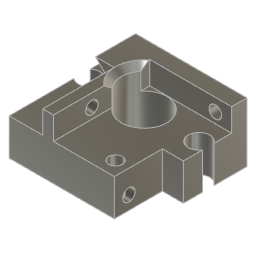
hotswap mx solderable v5 (Autodesk Fusion 360 design; units mm, degrees)
Autodesk Fusion 360 part; units mm, degrees
note: some values were not read from the file. Chosen so that the rebuilt part matches the saved one: which bodies a step acts on; which face or edge a step refers to. Set by a fixed rule: which sketch regions a step uses.
sketch "body" plane through (0, 0, 0) normal (0, 0, 1) x (1, 0, 0)
  circle A0 centre (0, 0) radius 2
  circle A1 centre (4.8, 0) radius 0.95
  circle A2 centre (-4.8, 0) radius 0.95
  circle A3 centre (2.6, -5.1) radius 0.6
  circle A4 centre (-3.8, -2.5) radius 0.6
  line L0 (-5.426, 3.3769) -> (5.6055, 3.3769)
  line L1 (5.6055, 3.3769) -> (5.6055, -6.3722)
  line L2 (5.6055, -6.3722) -> (-5.426, -6.3722)
  line L3 (-5.426, -6.3722) -> (-5.426, 3.3769)
  line L4 (5.6055, -6.3722) -> (3.771, -6.3722)
  line L5 (3.771, -6.3722) -> (3.771, -2.1749)
  line L6 (3.771, -2.1749) -> (5.6055, -2.1749)
  line L7 (5.6055, -2.1749) -> (5.6055, -6.3722)
  line L8 (-5.426, 3.3769) -> (-8.926, 3.3769)
  line L9 (-8.926, 3.3769) -> (-8.926, -1.5107)
  line L10 (-8.926, -1.5107) -> (-5.426, -1.5107)
  line L11 (-5.426, -1.5107) -> (-5.426, 3.3769)
  line L12 (5.6055, 3.3769) -> (9.1055, 3.3769)
  line L13 (9.1055, 3.3769) -> (9.1055, -1.4945)
  line L14 (9.1055, -1.4945) -> (5.6055, -1.4945)
  line L15 (5.6055, -1.4945) -> (5.6055, 3.3769)
  line L16 (-8.926, -1.5107) -> (-7.426, -1.5107)
  line L17 (-7.426, -1.5107) -> (-7.426, -5.9318)
  line L18 (-7.426, -5.9318) -> (-8.926, -5.9318)
  line L19 (-8.926, -5.9318) -> (-8.926, -1.5107)
  line L20 (9.1055, -1.4945) -> (7.6055, -1.4945)
  line L21 (7.6055, -1.4945) -> (7.6055, -5.9318)
  line L22 (7.6055, -5.9318) -> (9.1055, -5.9318)
  line L23 (9.1055, -5.9318) -> (9.1055, -1.4945)
  line L24 (6.7444, -1.4945) -> (6.7444, 3.3769)
  line L25 (-6.3235, -1.5107) -> (-6.3235, 3.3769)
  dimension "d1" = 4
  dimension "d2" = 1.9
  dimension "d3" = 1.9
  dimension "d4" = 4.8
  dimension "d5" = 4.8
  dimension "d6" = 1.2
  dimension "d7" = 1.2
  dimension "d8" = 3.8
  dimension "d9" = 2.5
  dimension "d10" = 5.1
  dimension "d11" = 2.6
  dimension "d84" = 6.3722
  dimension "d85" = 5.426
  dimension "d95" = 3.5
  dimension "d96" = 3.5
  dimension "d103" = 1.5
  dimension "d104" = 1.5
  constraint coincident A0.centre origin
  constraint horizontal L0
  constraint vertical L1
  constraint horizontal L2
  constraint vertical L3
  constraint horizontal L4
  constraint vertical L5
  constraint horizontal L6
  constraint vertical L7
  constraint horizontal A0.centre A2.centre
  constraint horizontal A0.centre A1.centre
  constraint horizontal L8
  constraint vertical L9
  constraint horizontal L10
  constraint vertical L11
  constraint horizontal L12
  constraint vertical L13
  constraint horizontal L14
  constraint vertical L15
  constraint horizontal L16
  constraint vertical L17
  constraint horizontal L18
  constraint vertical L19
  constraint horizontal L20
  constraint vertical L21
  constraint horizontal L22
  constraint vertical L23
  constraint coincident L17.end L22
  constraint coincident L14 L24.start
  constraint coincident L12 L24.end
  constraint perpendicular L12 L24
  constraint coincident L8 L25.end
  constraint perpendicular L8 L25
  constraint coincident L10 L25.start
  measures "d1" diameter of A0
  measures "d2" diameter of A1
  measures "d3" diameter of A2
  measures "d4" horizontal distance of A0.centre A2.centre
  measures "d5" horizontal distance of A0.centre A1.centre
  measures "d6" diameter of A3
  measures "d7" diameter of A4
  measures "d8" horizontal distance of A0.centre A4.centre
  measures "d9" vertical distance of A0.centre A4.centre
  measures "d10" vertical distance of A0.centre A3.centre
  measures "d11" horizontal distance of A0.centre A3.centre
  measures "d84" distance of A0.centre L2
  measures "d85" distance of A0.centre L3
  measures "d95" distance of L0.start L8.end
  measures "d96" distance of L0.end L12.end
  measures "d103" distance of L9.end L16.end
  measures "d104" distance of L13.end L20.end
extrude "Extrude1" add sketch "body" along normal blind 3.2 contours A1 L1 L12 L14 L15 L24 | A1 A2 L0 L1 L2 L3 L5 L6 L11 L15 | A2 L3 L8 L10 L11 L25 | L12 L13 L14 L20 L24 | L8 L9 L10 L16 L25 | L14 L20 L21 L22 L23 | L10 L16 L17 L18 L19 makes body 1
sketch "side holes" plane through (0, 0, 0) normal (1, 0, 0) x (0, 1, 0)
  circle A0 centre (-5.1, 1.1729) radius 0.55
  circle A1 centre (-2.5, 1.1388) radius 0.55
  point P0 (-2.5, 0)
  point P1 (-5.1, 0)
  dimension "d14" = 1.1
  dimension "d15" = 1.1
  constraint vertical P1 A0.centre
  constraint vertical P0 A1.centre
  measures "d14" diameter of A0
  measures "d15" diameter of A1
extrude "Extrude2" cut sketch "side holes" along normal up to surface (9.197 mm away) from surface at -5.426 bodies 1
sketch "2nd layer" plane through (0, 0, 3.2) normal (0, 0, 1) x (-1, 0, 0)
  circle A0 centre (3.8, 2.5) radius 0.6
  circle A1 centre (0, 0) radius 2
  circle A2 centre (-2.6, 5.1) radius 0.6
  line L0 (-3.771, 6.3722) -> (-3.771, 2.1749)
  line L1 (-3.771, 2.1749) -> (-5.6055, 2.1749)
  line L2 (-5.6055, 2.1749) -> (-5.6055, 1.4945)
  line L3 (-9.1055, -3.3769) -> (8.926, -3.3769)
  line L4 (5.426, 1.5107) -> (5.426, 6.3722)
  line L5 (5.426, 6.3722) -> (-3.771, 6.3722)
  line L6 (-9.1055, -3.3769) -> (-2.7206, -3.3769)
  line L7 (-9.1055, -0.9358) -> (-9.1055, -3.3769)
  line L8 (-5.6055, -2.0433) -> (1.5542, -2.0433)
  line L9 (1.5542, -2.0433) -> (1.5542, -3.3769)
  line L10 (1.5542, -3.3769) -> (-5.6055, -3.3769)
  line L11 (-5.6055, -3.3769) -> (-5.6055, -2.0433)
  line L12 (5.426, -3.3769) -> (4.4901, -3.3769)
  line L13 (4.4901, -3.3769) -> (4.4901, 6.3722)
  line L14 (4.4901, 6.3722) -> (5.426, 6.3722)
  line L15 (5.426, 6.3722) -> (5.426, -3.3769)
  line L16 (1.5542, 6.3722) -> (2.4901, 6.3722)
  line L17 (2.4901, 6.3722) -> (2.4901, -3.3769)
  line L18 (2.4901, -3.3769) -> (1.5542, -3.3769)
  line L19 (1.5542, -3.3769) -> (1.5542, 6.3722)
  line L20 (-9.1055, -3.3769) -> (8.926, -3.3769)
  line L21 (-2.7206, -3.3769) -> (-2.7206, -2.0433)
  line L22 (2.4901, 1.7119) -> (1.5542, 1.7119)
  circle A3 centre (-4.8, 0) radius 0.95
  circle A4 centre (4.8, 0) radius 0.95
  line L23 (-5.6055, 1.4945) -> (-7.6055, 1.4945)
  line L24 (-9.1055, 5.9318) -> (-9.1055, -3.3769)
  line L25 (8.926, -3.3769) -> (8.926, 5.9318)
  line L26 (7.426, 1.5107) -> (5.426, 1.5107)
  line L27 (5.426, 6.3722) -> (-3.771, 6.3722)
  line L28 (-7.6055, 1.4945) -> (-7.6055, 5.9318)
  line L29 (-7.6055, 5.9318) -> (-9.1055, 5.9318)
  line L30 (8.926, 5.9318) -> (7.426, 5.9318)
  line L31 (7.426, 5.9318) -> (7.426, 1.5107)
  dimension "d39" = 2
  constraint horizontal L6
  constraint vertical L7
  constraint coincident L3.start L6.start
  constraint horizontal L8
  constraint vertical L9
  constraint horizontal L10
  constraint vertical L11
  constraint horizontal L12
  constraint vertical L13
  constraint horizontal L14
  constraint vertical L15
  constraint coincident L4 L12.start
  constraint horizontal L16
  constraint vertical L17
  constraint horizontal L18
  constraint vertical L19
  constraint equal L14 L16
  constraint coincident L18 L3.end
  constraint coincident L12 L3.end
  constraint coincident L9 L16.start
  constraint coincident L10 L6.end
  constraint coincident L8 L21.end
  constraint perpendicular L8 L21
  constraint coincident L17 L22.start
  constraint coincident L19 L22.end
  constraint perpendicular L19 L22
  constraint coincident L6.end L21.start
  measures "d39" distance of L13 L17
extrude "Extrude3" add sketch "2nd layer" along normal blind 2 contours A1 L3 L9 L17 L18 L19 L20 L22 | L5 L16 L17 L19 L22 L27 | L3 L8 L9 L10 L19 L20 L21 | L3 L6 L8 L10 L11 L20 L21 bodies 1
sketch "diode fitting" plane through (0, 0, 0) normal (0, 1, 0) x (1, 0, 0)
  circle A0 centre (4.1902, -4.093) radius 0.55
  dimension "d21" = 1.1
  measures "d21" diameter of A0
extrude "Extrude4" cut sketch "diode fitting" against normal up to surface (5.5518 mm away) from surface at 3.3769 bodies 1
sketch "side hole for second layer" plane through (0, 0, 0) normal (1, 0, 0) x (0, 1, 0)
  circle A0 centre (-3.011, 4.093) radius 0.55
  point P0 (-2.5, 1.1388)
  dimension "d25" = 1.1
  measures "d25" diameter of A0
extrude "Extrude5" cut sketch "side hole for second layer" along normal up to surface (3.8718 mm away) from surface at -5.426 bodies 1
extrude "Extrude6" add sketch "side holes" against normal blind 1 from surface at 3.771 contours A1 bodies 1
extrude "Extrude7" add sketch "side holes" along normal blind 1.626 from surface at -5.426 contours A0 bodies 1
sketch "Sketch6" plane through (0, 0, 3.2) normal (0, 0, 1) x (-1, 0, 0)
  line L0 (1.5542, 6.3722) -> (-3.771, 6.3722)
  line L1 (-3.771, 6.3722) -> (-3.771, 2.1749)
  line L2 (-5.6055, -2.0433) -> (1.5542, -2.0433)
  circle A0 centre (-2.6, 5.1) radius 0.6
  line L3 (5.426, -3.3769) -> (-9.1055, -3.3769)
  line L4 (-9.1055, -3.3769) -> (-9.1055, 2.1749)
  line L5 (-9.1055, 2.1749) -> (5.426, 2.1749)
  line L6 (5.426, 2.1749) -> (5.426, -3.3769)
  line L7 (5.426, 2.1749) -> (-3.771, 2.1749)
  line L8 (-3.771, 2.1749) -> (-3.771, 6.3722)
  line L9 (-3.771, 6.3722) -> (5.426, 6.3722)
  line L10 (5.426, 6.3722) -> (5.426, 2.1749)
  circle A1 centre (3.8, 2.5) radius 0.6
  line L11 (-3.771, 2.1749) -> (-5.6055, 2.1749)
  line L12 (-5.6055, 2.1749) -> (-5.6055, 1.4945)
  circle A2 centre (0, 0) radius 2
  line L13 (-5.6055, -3.3769) -> (-5.6055, -2.0433)
  line L14 (-5.6055, 1.4945) -> (-7.6055, 1.4945)
  line L15 (-9.1055, 5.9318) -> (-9.1055, -3.3769)
  line L16 (-9.1055, -3.3769) -> (-5.6055, -3.3769)
  arc A3 (1.5542, 1.2588) -> (1.5542, -1.2588) centre (0, 0) ccw
  circle A4 centre (-4.8, 0) radius 0.95
  line L17 (1.5542, -2.0433) -> (1.5542, -1.2588)
  arc A5 (1.5542, 1.2588) -> (1.5542, -1.2588) centre (0, 0) ccw
  line L18 (1.5542, 1.2588) -> (1.5542, 6.3722)
  line L19 (-7.6055, 1.4945) -> (-7.6055, 5.9318)
  line L20 (-7.6055, 5.9318) -> (-9.1055, 5.9318)
  point P0 (5.426, -3.3769)
  point P1 (-9.1055, -3.3769)
  constraint horizontal L3
  constraint vertical L4
  constraint horizontal L5
  constraint vertical L6
  constraint coincident L3 P0
  constraint coincident L4 P1
  constraint coincident L6 P0
  constraint horizontal L7
  constraint vertical L8
  constraint horizontal L9
  constraint vertical L10
  constraint coincident L0.end L1.start
sketch "Sketch11" plane through (0, 3.3769, 0) normal (0, 1, 0) x (-1, 0, 0)
  line L0 (-9.1055, 0) -> (8.926, 0)
  line L1 (2.4901, 3.2) -> (2.4901, 5.2)
  line L2 (2.4901, 5.2) -> (-5.6055, 5.2)
  line L3 (2.4901, 5.2) -> (4.1182, 5.2)
  line L4 (4.1182, 5.2) -> (2.4901, 3.572)
  line L5 (8.926, 0) -> (8.926, 3.2)
  line L6 (8.926, 3.2) -> (2.4901, 3.2)
  line L7 (-5.6055, 3.2) -> (-9.1055, 3.2)
  line L8 (-9.1055, 3.2) -> (-9.1055, 0)
  circle A0 centre (-4.1902, 4.093) radius 0.55
  line L9 (-5.6055, 5.2) -> (-5.6055, 3.2)
  dimension "d91" = 45
  constraint coincident L1.end L2.start
  constraint perpendicular L1 L3
  constraint coincident L1 L4.end
  measures "d91" angle of L3 L4
extrude "Extrude17" add sketch "Sketch11" against normal blind 3.5 contours L1 L3 L4 bodies 1
extrude "Extrude18" cut sketch "body" along normal blind 2.5 contours L12 L13 L14 L20 L24 | L8 L9 L10 L16 L25 | L14 L20 L21 L22 L23 | L10 L16 L17 L18 L19 bodies 1
chamfer "Chamfer12" distance 0.5 angle 45 1 edges at (-2, 0, 5.2) on bodies 1
sketch "Sketch12" plane through (0, 3.3769, 0) normal (0, 1, 0) x (-1, 0, 0)
  line L0 (-6.7444, 2.5) -> (-6.7444, 0)
  line L1 (-6.7444, 0) -> (6.3235, 0)
  line L2 (6.3235, 0) -> (6.3235, 2.5)
  line L3 (6.3235, 2.5) -> (8.926, 2.5)
  line L4 (8.926, 2.5) -> (8.926, 3.2)
  line L5 (8.926, 3.2) -> (2.4901, 3.2)
  line L6 (2.4901, 3.2) -> (2.4901, 3.572)
  line L7 (2.4901, 3.572) -> (4.1182, 5.2)
  line L8 (4.1182, 5.2) -> (-5.6055, 5.2)
  line L9 (-5.6055, 5.2) -> (-5.6055, 3.2)
  line L10 (-5.6055, 3.2) -> (-9.1055, 3.2)
  line L11 (-9.1055, 3.2) -> (-9.1055, 2.5)
  line L12 (-9.1055, 2.5) -> (-6.7444, 2.5)
  circle A0 centre (-4.1902, 4.093) radius 0.55
  circle A1 centre (-6.7444, 1.25) radius 1.0614
  circle A2 centre (6.3235, 1.25) radius 1.1016
  constraint midpoint L0 A1.centre
  constraint midpoint L2 A2.centre
extrude "Extrude19" cut sketch "Sketch12" against normal blind 5.9 contours L0 A1 | L2 A2 | L2 A2 picked at (-6.3627, 1.5067) bodies 1
split "Split1" by plane through (-5.426, 0, 0) normal (-1, 0, 0) bodies 1 makes body 2 at (-7.3547, 0.7107, 3.2) makes body 3 at (-5.8397, 0.6161, 0.2603)
split "Split2" by plane through (5.6055, -1.4945, 0) normal (1, 0, 0) bodies 1 makes body 4 at (7.4747, 0.7148, 3.2)
hidden bodies 2 3 4
equation "d3 = d2"
equation "d5 = d4"
equation "d6 = d7"
named bodies: "mx bottom  fixable", "mx bottom  fixable (1)", "mx bottom  fixable (2)", "mx bottom  fixable (3)"
